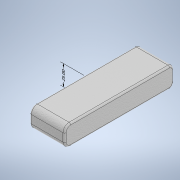
# Autodesk Inventor part: LiPo
Saved by Autodesk Inventor 2020.4 (Build 244396000, 396)
## iProperties
Created: 2021-04-27
Part Number: LiPo
Material: PPS Plastic
Document SubType Name: Modeling
Designer: armin
Density: 1.637 g/cm^3
Appearance: Coarse Textured - White
Author: armin
Autodesk Inventor part; units mm, degrees
ref_plane "YZ Plane" through (0, 0, 0) normal (1, 0, 0) x (0, 1, 0)
ref_plane "XZ Plane" through (0, 0, 0) normal (0, 1, 0) x (-1, 0, 0)
ref_plane "XY Plane" through (0, 0, 0) normal (0, 0, 1) x (1, 0, 0)
sketch "Sketch2" plane through (0, 0, 0) normal (0, 1, 0) x (-1, 0, 0)
  line L0 (0, 0) -> (43, 0)
  line L1 (43, 0) -> (43, -135)
  line L2 (43, -135) -> (0, -135)
  line L3 (0, -135) -> (0, 0)
  dimension "d0" = 43
  dimension "d1" = 135
  constraints: 8 end point, 2 parallel, 1 horizontal, 1 perpendicular
  measures "d0" distance of L1.end L2.end
  measures "d1" distance of L0.end L1.end
extrude "Extrusion1" add sketch "Sketch2" along normal blind 25
fillet "Fillet1" radius 7.5 2 edges at (-21.5, 25, 0) (-21.5, 0, 0)
fillet "Fillet2" radius 5.25 2 edges at (-21.5, 25, -135) (-21.5, 0, -135)
fillet "Fillet3" radius 2 16 edges at (0, 23.4623, -133.4623) (0, 12.5, -135) (0, 1.5377, -133.4623) (0, 0, -68.625) (0, 2.1967, -2.1967) (0, 12.5, 0) (0, 22.8033, -2.1967) (0, 25, -68.625) (-43, 22.8033, -2.1967) (-43, 12.5, 0) (-43, 2.1967, -2.1967) (-43, 0, -68.625) (-43, 1.5377, -133.4623) (-43, 12.5, -135) (-43, 23.4623, -133.4623) (-43, 25, -68.625)
body "Solid1"
